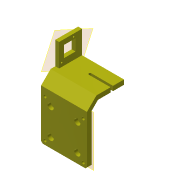
# Autodesk Inventor part: cellSTORM_v5_laserstage
Saved by Autodesk Inventor 2022 (Build 260153000, 153)
## iProperties
Created: 2020-04-25
Part Number: cellSTORM_v5_laserstage
Material: Generic
Document SubType Name: Modeling
Designer: diederichbenedict
Density: 1 g/cm^3
Appearance: Yellow
Author: diederichbenedict
Autodesk Inventor part; units mm, degrees
ref_plane "YZ Plane" through (0, 0, 0) normal (1, 0, 0) x (0, 1, 0)
ref_plane "XZ Plane" through (0, 0, 0) normal (0, 1, 0) x (-1, 0, 0)
ref_plane "XY Plane" through (0, 0, 0) normal (0, 0, 1) x (1, 0, 0)
ref_plane "Work Plane1" through (0, 0, 0) normal (0, 0, 1) x (1, 0, 0)
ref_plane "Work Plane2" through (-30, -30, 6) normal (0, 0, -1) x (0, 1, 0)
sketch "Sketch1" plane through (0, 0, 0) normal (0, 0, 1) x (1, 0, 0)
  circle A0 centre (-25, 0) radius 1.95 projected
  circle A1 centre (0, -25) radius 1.95 projected
  circle A2 centre (25, -25) radius 1.95 projected
  circle A3 centre (-25, 25) radius 1.95 projected
  circle A4 centre (25, 25) radius 1.95 projected
  circle A5 centre (-25, -25) radius 1.95 projected
  circle A6 centre (0, 25) radius 1.95 projected
  circle A7 centre (25, 0) radius 1.95 projected
  line L0 (-30, -28) -> (-28, -30) projected
  line L1 (-28, -30) -> (28, -30) projected
  line L2 (28, -30) -> (30, -28) projected
  line L3 (30, -28) -> (30, 28) projected
  line L4 (30, 28) -> (28, 30) projected
  line L5 (28, 30) -> (-28, 30) projected
  line L6 (-28, 30) -> (-30, 28) projected
  line L7 (-30, 28) -> (-30, -28) projected
  line L8 (43, -44) -> (44, -44) projected
  line L9 (76, -44) -> (145, -44) construction
  point P0 (0, 0)
  point P1 (30, 25)
  constraints: 2 end point, 1 horizontal, 1 point on line
extrude "Extrusion1" add sketch "Sketch1" along normal up to surface (6 mm away) contours A0 | A1 | A2 | A3 | A4 | A5 | A6 | A7 | L7 L6 L5 L4 L3 L2 L1 L0
sketch "Sketch2" plane through (-28, 30, 6) normal (0, 0, 1) x (1, 0, 0)
  circle A0 centre (10.5, -12.5) radius 1.95 projected
  circle A1 centre (10.5, -47.5) radius 1.95 projected
  circle A2 centre (45.5, -47.5) radius 1.95 projected
  circle A3 centre (45.5, -12.5) radius 1.95 projected
  point P0 (28, -30)
hole "Hole1" at (-17.5, -17.5, 6) at (17.5, -17.5, 6) at (17.5, 17.5, 6) at (-17.5, 17.5, 6) direction (0, 0, -1) diameter 4 end through all counterbore diameter 8 counterbore depth 4.5
sketch "Sketch10" plane through (0, 0, 0) normal (0, 0, -1) x (-1, 0, 0)
  circle A0 centre (-25, 25) radius 2.325 projected
  circle A1 centre (-25, -25) radius 2.325 projected
  circle A2 centre (25, 25) radius 2.325 projected
  circle A3 centre (25, -25) radius 2.325 projected
  circle A4 centre (25, -25) radius 2.325 projected
  point P0 (0, 0)
hole "Hole3" at (-25, 25, 0) at (25, 25, 0) at (-25, -25, 0) at (25, -25, 0) direction (0, 0, 1) diameter 3.8 depth 20 tip angle 118
sketch "Skizze13" plane through (30, -28, 0) normal (1, 0, 0) x (0, 0, -1)
  line L0 (0, 56) -> (-6, 56) projected
  line L1 (-6, 56) -> (-6, 58) projected
  line L2 (0, 56) -> (0, 58) projected
  line L3 (0, 58) -> (-6, 58) projected
  line L4 (-6, 58) -> (-6, 63)
  line L5 (-6, 63) -> (6.4834, 75.4834)
  line L6 (10.5521, 75.4834) -> (12.5521, 75.4834)
  line L7 (0, 58) -> (0, 61)
  line L8 (0, 61) -> (8.4834, 69.4834)
  line L9 (8.4834, 69.4834) -> (42.5521, 69.4834)
  line L10 (42.5521, 69.4834) -> (42.5521, 75.4834)
  line L11 (42.5521, 75.4834) -> (6.4834, 75.4834)
  line L12 (42.5521, 75.4834) -> (42.5521, 107.4834)
  point P0 (0, 28)
  dimension "d43" = 5
  dimension "d44" = 135
  dimension "d45" = 135
  dimension "d46" = 0
  dimension "d49" = 6
  constraints: 18 end point, 3 perpendicular, 3 vertical, 1 horizontal, 1 point on line, 4 other
  measures "d43" distance of L1.end L4.end
  measures "d44" angle of L4 L5
  measures "d45" angle of L7 L8
  measures "d46" distance from line of L12.start L10
  measures "d49" distance from line of L9 L6.end
extrude "Extrusion10" add sketch "Skizze13" against normal up to surface (60 mm away)
ref_plane "Arbeitsebene4" through (-30, 57.7593, -26.2973) normal (1, 0, 0) x (0, -0.9086751, 0.417504)
sketch "Skizze14" plane through (-30, -28, 0) normal (-1, 0, 0) x (0, 0, 1)
  circle A0 centre (-16.0521, 80.4834) radius 1
  circle A1 centre (-31.5521, 101.9834) radius 1
  circle A2 centre (-36.5521, 73.9834) radius 1
  line L0 (-6.4834, 75.4834) -> (-42.5521, 75.4834) projected
  line L1 (-42.5521, 69.4834) -> (-42.5521, 75.4834) projected
  line L2 (-42.5521, 75.4834) -> (-12.5521, 75.4834)
  line L3 (-12.5521, 75.4834) -> (-12.5521, 105.4834)
  line L4 (-12.5521, 105.4834) -> (-42.5521, 105.4834)
  line L5 (-42.5521, 105.4834) -> (-42.5521, 75.4834)
  circle A3 centre (-26.5521, 91.4834) radius 2.6486
  line L6 (-34.0521, 83.9834) -> (-19.0521, 83.9834)
  line L7 (-19.0521, 83.9834) -> (-19.0521, 98.9834)
  line L8 (-19.0521, 98.9834) -> (-34.0521, 98.9834)
  line L9 (-34.0521, 98.9834) -> (-34.0521, 83.9834)
  line L10 (-34.0521, 83.9834) -> (-19.0521, 98.9834) construction
  line L11 (-19.0521, 83.9834) -> (-34.0521, 98.9834) construction
  point P0 (0, 28)
  point P1 (-12.5521, 75.4834)
  dimension "d50" = 30
  dimension "d51" = 30
  dimension "d52" = 15
  dimension "d53" = 15
  constraints: 20 end point, 4 centre point, 4 parallel, 2 horizontal, 2 midpoint, 2 perpendicular, 8 other
  measures "d50" distance of L4.end L3.end
  measures "d51" distance of L3.end L2.end
  measures "d52" distance of L8.end L7.end
  measures "d53" distance of L7.end L6.end
extrude "Extrusion11" add sketch "Skizze14" against normal blind 5 contours L0 L5 L4 L3
sketch "Skizze15" plane through (30, 47.4834, -6.4834) normal (0, 1, 0) x (1, 0, 0)
  circle A0 centre (-15, 20.0687) radius 1.4
  line L0 (2.6067, 20.0687) -> (-28.3951, 20.0687) construction
  line L1 (2.6067, 21.6687) -> (-28.3951, 21.6687)
  line L2 (-28.3951, 18.4687) -> (2.6067, 18.4687)
  arc A1 (2.6067, 18.4687) -> (2.6067, 21.6687) centre (2.6067, 20.0687) ccw
  arc A2 (-28.3951, 21.6687) -> (-28.3951, 18.4687) centre (-28.3951, 20.0687) ccw
  point P0 (-30, -6.4834)
  point P1 (-12.8942, 20.0687)
  dimension "d56" = 3.2
  constraints: 8 end point, 4 point on circle, 4 tangent, 3 centre point, 1 horizontal, 1 midpoint, 1 parallel, 1 point on line, 2 other
  measures "d56" diameter of A2
extrude "Extrusion12" cut sketch "Skizze15" against normal through all contours A0 | A1 L2 A2 L1
body "Solid1"
